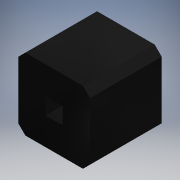
# Autodesk Inventor part: Kontakthalter
Saved by Autodesk Inventor 2019 (Build 230136000, 136)
## iProperties
Created: 2019-03-11
Part Number: Kontakthalter
Material: PBT-Kunststoff
Document SubType Name: Modeling
Designer: manue
Density: 1.31 g/cm^3
Appearance: Glatt - Schwarz
Author: manue
Autodesk Inventor part; units mm, degrees
ref_plane "YZ Plane" through (0, 0, 0) normal (1, 0, 0) x (0, 1, 0)
ref_plane "XZ Plane" through (0, 0, 0) normal (0, 1, 0) x (-1, 0, 0)
ref_plane "XY Plane" through (0, 0, 0) normal (0, 0, 1) x (1, 0, 0)
ref_plane "Arbeitsebene1" through (0, 0, 0) normal (0, 0, 1) x (1, 0, 0)
sketch "Skizze1" plane through (0, 0, 0) normal (0, 0, 1) x (1, 0, 0)
  line L0 (0, 0) -> (-0.6, 0) projected
  line L1 (0, 0.6) -> (0, 0) projected
  line L2 (-0.6, 0) -> (-0.6, 0.6) projected
  line L3 (-0.6, 0.6) -> (0, 0.6) projected
  line L4 (-1.57, -0.97) -> (0.97, -0.97)
  line L5 (0.97, -0.97) -> (0.97, 1.57)
  line L6 (0.97, 1.57) -> (-1.57, 1.57)
  line L7 (-1.57, 1.57) -> (-1.57, -0.97)
  line L8 (-1.57, -0.97) -> (0.97, 1.57) construction
  line L9 (0.97, -0.97) -> (-1.57, 1.57) construction
  point P0 (-0.3, 0.3)
  point P1 (-0.3, 0.3)
  point P2 (-0.6, 0.3)
  point P3 (-0.3, -0.97)
  point P4 (-0.3, 0)
  dimension "d0" = 2.54
  constraints: 12 end point, 6 midpoint, 2 parallel, 2 perpendicular, 1 horizontal, 1 horizontal alignment, 1 vertical alignment
  measures "d0" distance of L4.end L5.end
extrude "Extrusion1" add sketch "Skizze1" along normal blind 2.54
chamfer "Fase1" distance 0.25 angle 45 4 edges at (-1.57, -0.97, 1.27) (0.97, -0.97, 1.27) (0.97, 1.57, 1.27) (-1.57, 1.57, 1.27)
